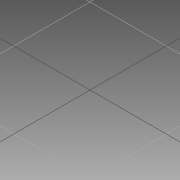
# Autodesk Inventor part: New Bot
Saved by Autodesk Inventor 2018 (Build 220112000, 112)
## iProperties
Created: 2017-12-11
Part Number: New Bot
Material: Generic
Document SubType Name: Modeling
Designer: Rus
Density: 1 g/cm^3
Appearance: Default
Author: Rus
Autodesk Inventor part; units mm, degrees
ref_plane "YZ Plane" through (0, 0, 0) normal (1, 0, 0) x (0, 1, 0)
ref_plane "XZ Plane" through (0, 0, 0) normal (0, 1, 0) x (-1, 0, 0)
ref_plane "Work Plane1" through (-109.2301, 56.494, 41.8932) normal (1, 0, 0) x (0, 1, 0)
sketch "Sketch1" plane through (-109.2301, 56.494, 41.8932) normal (1, 0, 0) x (0, 1, 0)
  line L0 (6.35, 0) -> (6.35, -6.35) projected
  line L1 (6.35, 0) -> (0, 0) projected
  line L2 (0, 0) -> (0, 9.525) projected
  line L3 (0, 9.525) -> (-3.175, 9.525) projected
  line L4 (-3.175, 9.525) -> (-3.175, 12.7) projected
  line L5 (-3.175, 12.7) -> (-6.35, 12.7) projected
  line L6 (-6.35, 12.7) -> (-6.35, -6.35) projected
  line L7 (-6.35, -6.35) -> (6.35, -6.35) projected
  line L8 (0, -6.35) -> (76.8547, -6.35) projected
  line L9 (76.8547, 0) -> (76.8547, -6.35) projected
  line L10 (76.8547, 0) -> (0, 0) projected
  line L11 (0, 0) -> (0, -6.35) projected
  point P0 (-56.494, -41.8932)
ref_plane "Work Plane2" through (-16.5927, 50.144, 35.5432) normal (-1, 0, 0) x (0, 0, 1)
extrude "Extrusion1" add sketch "Sketch1" along normal up to surface (92.6375 mm away) contours L11 L7 L6 L5 L4 L3 L2
body "Solid1"
